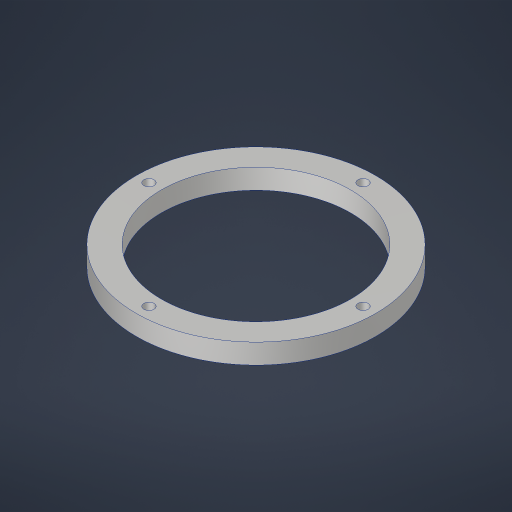
# Autodesk Inventor part: 4in LS-002
Saved by Autodesk Inventor 2023.4 (Build 274418000, 418)
## iProperties
Created: 2025-02-23
Part Number: 4in LS-002
Material: Aluminum 6061
Document SubType Name: Modeling
Designer: brand
Density: 2.7 g/cm^3
Appearance: Aluminum - Flat
Catalog Web Link: https://www.amazon.com/Aluminium-Turntable-Bearing-Rotating-Hardware/dp/B08CSMYXFV/ref=sr_1_4_sspa?dib=eyJ2IjoiMSJ9._dIJFbhkyI92XmDmKNkxFgU_0ePHUSC9YqSv3sFBVjlsdRyExycsbXiQU_MUmMUvJGy9GCAPT9QtxClaBTku0FbfhZoCtIpOYngGBTnJo919GddPBDS83ooZRsxJG5R7jq3cNUDygyRS_OmJipfkoM5OCq8T20qhxkRWpoecfTOp-jOGMSp8e54UpLORAgNJtiqEyScbtuTVsJE3J9O2aar2usHcvoaSkqYkZJUQvearKUFKK2c7Wpxg1pH32h2YCQUZluVIHso0mULp-QWUF_UNj0rclYvDnB-_XJVLeZI.44kslggF-zdLCPfpDMEyn6Enj3QOh1QtcF3QqGoJ9Ac&dib_tag=se&keywords=mini%2Blazy%2Bsusan&qid=1740338553&sr=8-4-spons&sp_csd=d2lkZ2V0TmFtZT1zcF9hdGY&th=1
Author: brand
Autodesk Inventor part; units mm, degrees
ref_plane "YZ Plane" through (0, 0, 0) normal (1, 0, 0) x (0, 1, 0)
ref_plane "XZ Plane" through (0, 0, 0) normal (0, 1, 0) x (-1, 0, 0)
ref_plane "XY Plane" through (0, 0, 0) normal (0, 0, 1) x (1, 0, 0)
sketch "Sketch1" plane through (0, 0, 0) normal (0, 1, 0) x (-1, 0, 0)
  circle A0 centre (0, 0) radius 35 construction
  circle A1 centre (0, 0) radius 47.5
  circle A2 centre (0, 0) radius 60
  line L0 (0, -35) -> (0, -60) construction
  point P0 (0, -47.5)
  dimension "d0" = 70
  dimension "d1" = 120
  constraints: 4 vertical alignment, 3 coincident, 2 end point, 1 midpoint, 1 vertical, 6 other
extrude "Extrusion1" add sketch "Sketch1" along normal mid plane 10
sketch "Sketch3" plane through (0, -5, 0) normal (0, -1, 0) x (1, 0, 0)
  circle A0 centre (0, 0) radius 47.5 construction
  circle A1 centre (0, 0) radius 60 construction
  circle A2 centre (0, 0) radius 47.5 construction
  line L0 (47.5, 0) -> (60, 0) construction
  circle A3 centre (0, 0) radius 47.5 construction
  circle A4 centre (0, 0) radius 60 construction
  point P0 (53.75, 0)
  constraints: 4 horizontal alignment, 2 end point, 1 horizontal, 1 midpoint, 3 other
hole "Hole2" at (53.75, -5, 0) direction (0, 1, 0) diameter 5.1054 end through all countersink diameter 9.779 countersink angle 82 clearance for "Flat Head Machine Screw (82)" size "#10" standard "Ansi Unified Screw Threads"
pattern_circular "Circular Pattern2" count 4 over 360 about axis through (0, 0, 0) along (0, 1, 0) of "Hole2"
body "Solid1"
